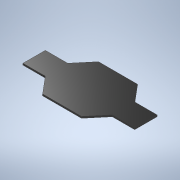
# Autodesk Inventor part: Base_plate
Saved by Autodesk Inventor 2020 (Build 240168000, 168)
## iProperties
Created: 2020-03-08
Part Number: Base_plate
Material: Acrylic, Clear
Document SubType Name: Modeling
Designer: 0x6f736f646f
Density: 1.19 g/cm^3
Appearance: Glossy - Black
Author: 0x6f736f646f
Autodesk Inventor part; units mm, degrees
ref_plane "YZ Plane" through (0, 0, 0) normal (1, 0, 0) x (0, 1, 0)
ref_plane "XZ Plane" through (0, 0, 0) normal (0, 1, 0) x (-1, 0, 0)
ref_plane "XY Plane" through (0, 0, 0) normal (0, 0, 1) x (1, 0, 0)
sketch "Sketch1" plane through (0, 0, 0) normal (0, 1, 0) x (-1, 0, 0)
  line L0 (-65.173, 0) -> (-134.827, 0)
  line L1 (-200, -30) -> (-200, -70)
  line L2 (-134.827, -100) -> (-65.173, -100)
  line L3 (0, -70) -> (0, -30)
  line L4 (0, -30) -> (-40, -30)
  line L5 (-40, -30) -> (-65.173, 0)
  line L6 (-134.827, 0) -> (-160, -30)
  line L7 (-160, -30) -> (-200, -30)
  line L8 (-134.827, -100) -> (-160, -70)
  line L9 (-160, -70) -> (-200, -70)
  line L10 (0, -70) -> (-40, -70)
  line L11 (-40, -70) -> (-65.173, -100)
  point P0 (0, 0)
  dimension "d13" = 130
  dimension "d14" = 130
  dimension "d15" = 130
  dimension "d17" = 130
  dimension "d18" = 40
  dimension "d19" = 40
  dimension "d20" = 40
  dimension "d21" = 40
  dimension "d22" = 40
  dimension "d23" = 30
  dimension "d24" = 30
  dimension "d25" = 200
  dimension "d26" = 30
  dimension "d27" = 30
  dimension "d28" = 40
  dimension "d29" = 69.654
  dimension "d30" = 69.654
  constraints: 24 end point, 4 point on line, 3 horizontal, 2 parallel, 1 perpendicular
  measures "d13" angle of L9 L8
  measures "d14" angle of L7 L6
  measures "d15" angle of L4 L5
  measures "d17" angle of L11 L10
  measures "d18" distance of L3.start L10.end
  measures "d19" distance of L3.end L4.end
  measures "d20" distance of L8.end L1.end
  measures "d21" distance of L6.end L1.start
  measures "d22" distance of L1.start L1.end
  measures "d23" distance between parallel lines of L9 L2
  measures "d24" distance between parallel lines of L0 L7
  measures "d25" distance between parallel lines of L1 L3
  measures "d26" distance between parallel lines of L10 L2
  measures "d27" distance between parallel lines of L4 L0
  measures "d28" distance of L3.start L3.end
  measures "d29" distance of L0.start L0.end
  measures "d30" distance of L2.start L2.end
extrude "Extrusion1" add sketch "Sketch1" along normal blind 3
body "Solid1"
